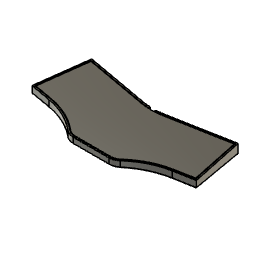
epssp75 case one-piece (Autodesk Fusion 360 design; units mm, degrees)
Autodesk Fusion 360 part; units mm, degrees
note: some values were not read from the file. Set by a fixed rule: which sketch regions a step uses.
(part 1 of 3)
sketch "Skizze1" plane through (0, 0, 0) normal (0, 0, 1) x (1, 0, 0)
  line L0 (-104.4744, 89.4694) -> (-90.6871, 87.0383)
  line L1 (-100.8347, 139.1928) -> (-114.622, 141.6239)
  line L2 (-84.0711, 124.5595) -> (-81.64, 138.3468)
  line L3 (-102.0433, 103.2567) -> (-104.4744, 89.4694)
  line L4 (-84.948, 119.5862) -> (-98.7353, 122.0173)
  line L5 (-88.256, 100.8256) -> (-102.0433, 103.2567)
  line L6 (-123.6691, 90.3154) -> (-109.8818, 87.8843)
  line L7 (-114.622, 141.6239) -> (-117.0531, 127.8365)
  line L8 (-81.64, 138.3468) -> (-95.4273, 140.7779)
  line L9 (-104.1427, 120.4322) -> (-117.93, 122.8633)
  line L10 (-107.4507, 101.6716) -> (-121.238, 104.1027)
  line L11 (-117.0531, 127.8365) -> (-103.2658, 125.4055)
  line L12 (-90.6871, 87.0383) -> (-88.256, 100.8256)
  line L13 (-97.8584, 126.9906) -> (-84.0711, 124.5595)
  line L14 (-109.8818, 87.8843) -> (-107.4507, 101.6716)
  line L15 (-103.2658, 125.4055) -> (-100.8347, 139.1928)
  line L16 (-121.238, 104.1027) -> (-123.6691, 90.3154)
  line L17 (-95.4273, 140.7779) -> (-97.8584, 126.9906)
  line L18 (-106.5738, 106.6449) -> (-104.1427, 120.4322)
  line L19 (-87.3791, 105.7989) -> (-84.948, 119.5862)
  line L20 (-98.7353, 122.0173) -> (-101.1664, 108.23)
  line L21 (-120.3611, 109.076) -> (-106.5738, 106.6449)
  line L22 (-101.1664, 108.23) -> (-87.3791, 105.7989)
  line L23 (-117.93, 122.8633) -> (-120.3611, 109.076)
  line L24 (-110.7587, 82.911) -> (-124.546, 85.3421)
  line L25 (-126.9771, 71.5548) -> (-113.1898, 69.1237)
  line L26 (-113.1898, 69.1237) -> (-110.7587, 82.911)
  line L27 (-124.546, 85.3421) -> (-126.9771, 71.5548)
  line L28 (-114.0667, 64.1504) -> (-127.854, 66.5815)
  line L29 (-130.2851, 52.7942) -> (-116.4978, 50.3631)
  line L30 (-116.4978, 50.3631) -> (-114.0667, 64.1504)
  line L31 (-127.854, 66.5815) -> (-130.2851, 52.7942)
  line L32 (-91.564, 82.065) -> (-105.3513, 84.4961)
  line L33 (-107.7824, 70.7088) -> (-93.9951, 68.2777)
  line L34 (-93.9951, 68.2777) -> (-91.564, 82.065)
  line L35 (-105.3513, 84.4961) -> (-107.7824, 70.7088)
  line L36 (-144.088, 84.2185) -> (-146.5191, 70.4311)
  line L37 (-165.2797, 73.7391) -> (-151.4924, 71.3081)
  line L38 (-154.8004, 52.5475) -> (-152.3693, 66.3348)
  line L39 (-140.78, 102.979) -> (-143.2111, 89.1917)
  line L40 (-166.1566, 68.7659) -> (-168.5877, 54.9786)
  line L41 (-126.1158, 105.5212) -> (-123.6847, 119.3086)
  line L42 (-144.8764, 108.8292) -> (-142.4453, 122.6166)
  line L43 (-168.5877, 54.9786) -> (-154.8004, 52.5475)
  line L44 (-126.9927, 100.548) -> (-140.78, 102.979)
  line L45 (-139.9031, 107.9523) -> (-126.1158, 105.5212)
  line L46 (-146.5191, 70.4311) -> (-132.7318, 68.0001)
  line L47 (-162.8486, 87.5265) -> (-165.2797, 73.7391)
  line L48 (-141.5684, 127.5898) -> (-139.1373, 141.3771)
  line L49 (-129.4238, 86.7607) -> (-126.9927, 100.548)
  line L50 (-123.6847, 119.3086) -> (-137.472, 121.7396)
  line L51 (-152.3693, 66.3348) -> (-166.1566, 68.7659)
  line L52 (-134.164, 140.5002) -> (-136.5951, 126.7129)
  line L53 (-139.1373, 141.3771) -> (-152.9246, 143.8082)
  line L54 (-136.5951, 126.7129) -> (-122.8078, 124.2818)
  line L55 (-143.2111, 89.1917) -> (-129.4238, 86.7607)
  line L56 (-158.6637, 111.2603) -> (-144.8764, 108.8292)
  line L57 (-161.9717, 92.4997) -> (-148.1844, 90.0687)
  line L58 (-149.0613, 85.0954) -> (-162.8486, 87.5265)
  line L59 (-142.4453, 122.6166) -> (-156.2326, 125.0476)
  line L60 (-148.1844, 90.0687) -> (-145.7533, 103.856)
  line L61 (-120.3767, 138.0691) -> (-134.164, 140.5002)
  line L62 (-155.3557, 130.0209) -> (-141.5684, 127.5898)
  line L63 (-156.2326, 125.0476) -> (-158.6637, 111.2603)
  line L64 (-137.472, 121.7396) -> (-139.9031, 107.9523)
  line L65 (-152.9246, 143.8082) -> (-155.3557, 130.0209)
  line L66 (-145.7533, 103.856) -> (-159.5406, 106.287)
  line L67 (-122.8078, 124.2818) -> (-120.3767, 138.0691)
  line L68 (-159.5406, 106.287) -> (-161.9717, 92.4997)
  line L69 (-132.7318, 68.0001) -> (-130.3007, 81.7874)
  line L70 (-151.4924, 71.3081) -> (-149.0613, 85.0954)
  line L71 (-130.3007, 81.7874) -> (-144.088, 84.2185)
  line L72 (-149.8271, 51.6706) -> (-136.0398, 49.2395)
  line L73 (-136.0398, 49.2395) -> (-133.6087, 63.0268)
  line L74 (-147.396, 65.4579) -> (-149.8271, 51.6706)
  line L75 (-133.6087, 63.0268) -> (-147.396, 65.4579)
  line L76 (-43.5823, 105.692) -> (-46.0133, 91.9047)
  line L77 (-28.918, 108.2342) -> (-26.4869, 122.0216)
  line L78 (-29.7949, 103.261) -> (-43.5823, 105.692)
  line L79 (-46.0133, 91.9047) -> (-32.226, 89.4737)
  line L80 (-42.7053, 110.6653) -> (-28.918, 108.2342)
  line L81 (-66.6215, 113.8162) -> (-80.4088, 116.2473)
  line L82 (-47.3313, 113.5119) -> (-44.9002, 127.2992)
  line L83 (-48.2082, 108.5386) -> (-61.9955, 110.9697)
  line L84 (-58.6875, 129.7302) -> (-61.1186, 115.9429)
  line L85 (-44.9002, 127.2992) -> (-58.6875, 129.7302)
  line L86 (-80.4088, 116.2473) -> (-82.8399, 102.46)
  line L87 (-32.226, 89.4737) -> (-29.7949, 103.261)
  line L88 (-69.0526, 100.0289) -> (-66.6215, 113.8162)
  line L89 (-64.4266, 97.1823) -> (-50.6393, 94.7513)
  line L90 (-82.8399, 102.46) -> (-69.0526, 100.0289)
  line L91 (-26.4869, 122.0216) -> (-40.2743, 124.4526)
  line L92 (-69.9295, 95.0556) -> (-83.7168, 97.4867)
  line L93 (-61.1186, 115.9429) -> (-47.3313, 113.5119)
  line L94 (-65.7446, 118.7895) -> (-63.3135, 132.5768)
  line L95 (-77.1008, 135.0079) -> (-79.5319, 121.2205)
  line L96 (-40.2743, 124.4526) -> (-42.7053, 110.6653)
  line L97 (-61.9955, 110.9697) -> (-64.4266, 97.1823)
  line L98 (-51.5162, 89.778) -> (-65.3035, 92.2091)
  line L99 (-63.3135, 132.5768) -> (-77.1008, 135.0079)
  line L100 (-79.5319, 121.2205) -> (-65.7446, 118.7895)
  line L101 (-50.6393, 94.7513) -> (-48.2082, 108.5386)
  line L102 (-83.7168, 97.4867) -> (-86.1479, 83.6994)
  line L103 (-68.6115, 73.4485) -> (-71.0426, 59.6612)
  line L104 (-72.3606, 81.2683) -> (-69.9295, 95.0556)
  line L105 (-57.2553, 57.2301) -> (-54.8242, 71.0174)
  line L106 (-86.1479, 83.6994) -> (-72.3606, 81.2683)
  line L107 (-53.9473, 75.9907) -> (-51.5162, 89.778)
  line L108 (-75.6686, 62.5077) -> (-73.2375, 76.295)
  line L109 (-54.8242, 71.0174) -> (-68.6115, 73.4485)
  line L110 (-65.3035, 92.2091) -> (-67.7346, 78.4218)
  line L111 (-67.7346, 78.4218) -> (-53.9473, 75.9907)
  line L112 (-71.0426, 59.6612) -> (-57.2553, 57.2301)
  line L113 (-87.0248, 78.7261) -> (-89.4559, 64.9388)
  line L114 (-73.2375, 76.295) -> (-87.0248, 78.7261)
  line L115 (-89.4559, 64.9388) -> (-75.6686, 62.5077)
  line L116 (-40.548, 85.3816) -> (-40.6913, 84.5691)
  line L117 (-38.9005, 60.0862) -> (-42.0814, 60.6471)
  line L118 (-43.9157, 76.735) -> (-48.5442, 77.5512)
  line L119 (-51.8862, 57.2734) -> (-52.1858, 55.5746)
  line L120 (-43.3968, 53.1872) -> (-43.2536, 53.9996)
  line L121 (-39.1207, 77.4381) -> (-35.9398, 76.8772)
  line L122 (-53.068, 57.4818) -> (-51.8862, 57.2734)
  line L123 (-34.7569, 75.1201) -> (-39.3855, 75.9362)
  line L124 (-46.6115, 61.4459) -> (-51.0136, 62.2221)
  line L125 (-40.0726, 53.4388) -> (-38.9005, 60.0862)
  line L126 (-43.6508, 78.2368) -> (-43.9157, 76.735)
  line L127 (-37.188, 61.3328) -> (-34.7569, 75.1201)
  line L128 (-48.9352, 80.9202) -> (-47.7534, 80.7118)
  line L129 (-48.0529, 79.0131) -> (-43.6508, 78.2368)
  line L130 (-50.9753, 63.7639) -> (-46.3467, 62.9477)
  line L131 (-43.2536, 53.9996) -> (-40.0726, 53.4388)
  line L132 (-41.8166, 62.1489) -> (-37.188, 61.3328)
  line L133 (-45.9962, 54.4833) -> (-46.1395, 53.6708)
  line L134 (-37.9486, 84.0855) -> (-37.8053, 84.898)
  line L135 (-35.9398, 76.8772) -> (-34.7677, 83.5246)
  line L136 (-47.1803, 83.9617) -> (-48.3621, 84.1701)
  line L137 (-34.7677, 83.5246) -> (-37.9486, 84.0855)
  line L138 (-37.8053, 84.898) -> (-40.548, 85.3816)
  line L139 (-51.0136, 62.2221) -> (-51.3132, 60.5233)
  line L140 (-39.3855, 75.9362) -> (-39.1207, 77.4381)
  line L141 (-46.1395, 53.6708) -> (-43.3968, 53.1872)
  line L142 (-48.5442, 77.5512) -> (-50.9753, 63.7639)
  line L143 (-46.8808, 85.6605) -> (-47.1803, 83.9617)
  line L144 (-52.1858, 55.5746) -> (-45.9962, 54.4833)
  line L145 (-48.3621, 84.1701) -> (-48.9352, 80.9202)
  line L146 (-42.0814, 60.6471) -> (-41.8166, 62.1489)
  line L147 (-52.4949, 60.7317) -> (-53.068, 57.4818)
  line L148 (-46.3467, 62.9477) -> (-46.6115, 61.4459)
  line L149 (-51.3132, 60.5233) -> (-52.4949, 60.7317)
  line L150 (-47.7534, 80.7118) -> (-48.0529, 79.0131)
  line L151 (-40.6913, 84.5691) -> (-46.8808, 85.6605)
  line L152 (0, 1.75) -> (0, 22.5)
  line L153 (15.275, 92.8) -> (16.1, 92.8)
  line L154 (8.525, 89.57) -> (15.275, 89.57)
  line L155 (13.55, 103.07) -> (10.25, 103.07)
  line L156 (-7, 88.1) -> (7, 88.1)
  line L157 (10.25, 101.87) -> (8.525, 101.87)
  line L158 (16.1, 92.8) -> (16.1, 95.585)
  line L159 (15.275, 101.87) -> (13.55, 101.87)
  line L160 (13.55, 101.87) -> (13.55, 103.07)
  line L161 (16.1, 95.585) -> (15.275, 95.585)
  line L162 (7, 88.1) -> (7, 92.8)
  line L163 (15.275, 95.585) -> (15.275, 101.87)
  line L164 (10.25, 103.07) -> (10.25, 101.87)
  line L165 (8.525, 101.87) -> (8.525, 97.4)
  line L166 (15.275, 89.57) -> (15.275, 92.8)
  line L167 (7, 97.4) -> (7, 102.1)
  line L168 (7, 92.8) -> (8.525, 92.8)
  line L169 (8.525, 92.8) -> (8.525, 89.57)
  line L170 (8.525, 97.4) -> (7, 97.4)
  line L171 (-8.525, 89.57) -> (-8.525, 92.8)
  line L172 (-7, 92.8) -> (-7, 88.1)
  line L173 (-16.1, 95.585) -> (-16.1, 92.8)
  line L174 (-15.275, 92.8) -> (-15.275, 89.57)
  line L175 (-7, 97.4) -> (-8.525, 97.4)
  line L176 (-15.275, 95.585) -> (-16.1, 95.585)
  line L177 (-15.275, 89.57) -> (-8.525, 89.57)
  line L178 (-8.525, 92.8) -> (-7, 92.8)
  line L179 (-10.25, 101.87) -> (-10.25, 103.07)
  line L180 (-13.55, 103.07) -> (-13.55, 101.87)
  line L181 (-8.525, 101.87) -> (-10.25, 101.87)
  line L182 (-13.55, 101.87) -> (-15.275, 101.87)
  line L183 (-15.275, 101.87) -> (-15.275, 95.585)
  line L184 (-8.525, 97.4) -> (-8.525, 101.87)
  line L185 (-10.25, 103.07) -> (-13.55, 103.07)
  line L186 (-7, 102.1) -> (-7, 97.4)
  line L187 (7, 102.1) -> (-7, 102.1)
  line L188 (-16.1, 92.8) -> (-15.275, 92.8)
  line L189 (-2.525, 121.15) -> (-16.525, 121.15)
  line L190 (-16.525, 121.15) -> (-16.525, 107.15)
  line L191 (-16.525, 107.15) -> (-2.525, 107.15)
  line L192 (-2.525, 107.15) -> (-2.525, 121.15)
  line L193 (16.525, 107.15) -> (16.525, 121.15)
  line L194 (2.525, 107.15) -> (16.525, 107.15)
  line L195 (16.525, 121.15) -> (2.525, 121.15)
  line L196 (2.525, 121.15) -> (2.525, 107.15)
  line L197 (7, 83.05) -> (-7, 83.05)
  line L198 (12.05, 83.05) -> (12.05, 69.05)
  line L199 (26.05, 69.05) -> (26.05, 83.05)
  line L200 (-7, 69.05) -> (7, 69.05)
  line L201 (12.05, 69.05) -> (26.05, 69.05)
  line L202 (-7, 83.05) -> (-7, 69.05)
  line L203 (7, 69.05) -> (7, 83.05)
  line L204 (26.05, 83.05) -> (12.05, 83.05)
  line L205 (-12.05, 83.05) -> (-26.05, 83.05)
  line L206 (-12.05, 69.05) -> (-12.05, 83.05)
  line L207 (-26.05, 83.05) -> (-26.05, 69.05)
  line L208 (-26.05, 69.05) -> (-12.05, 69.05)
  line L209 (-26.05, 50) -> (-12.05, 50)
  line L210 (-12.05, 64) -> (-26.05, 64)
  line L211 (-12.05, 50) -> (-12.05, 64)
  line L212 (7, 64) -> (-7, 64)
  line L213 (-26.05, 64) -> (-26.05, 50)
  line L214 (-7, 64) -> (-7, 50)
  line L215 (26.05, 64) -> (12.05, 64)
  line L216 (7, 50) -> (7, 64)
  line L217 (12.05, 50) -> (26.05, 50)
  line L218 (26.05, 50) -> (26.05, 64)
  line L219 (12.05, 64) -> (12.05, 50)
  line L220 (-7, 50) -> (7, 50)
  line L221 (-108.7367, 55.9946) -> (-113.525, 42.8389)
  line L222 (-95.581, 51.2064) -> (-108.7367, 55.9946)
  line L223 (-100.3693, 38.0507) -> (-95.581, 51.2064)
  line L224 (-113.525, 42.8389) -> (-100.3693, 38.0507)
  line L225 (-64.2085, 29.3272) -> (-62.5935, 32.1245)
  line L226 (-62.5935, 32.1245) -> (-61.879, 31.712)
  line L227 (-87.658, 49.8113) -> (-88.3725, 50.2238)
  line L228 (-89.765, 47.812) -> (-89.0505, 47.3995)
  line L229 (-84.8199, 41.2272) -> (-83.2049, 44.0245)
  line L230 (-68.4391, 35.4995) -> (-70.0541, 32.7022)
  line L231 (-84.2342, 39.1916) -> (-72.1098, 32.1916)
  line L232 (-90.6655, 44.6022) -> (-84.8199, 41.2272)
  line L233 (-88.3725, 50.2238) -> (-89.765, 47.812)
  line L234 (-60.4865, 34.1238) -> (-61.201, 34.5363)
  line L235 (-77.2342, 51.316) -> (-79.5842, 47.2457)
  line L236 (-58.0585, 39.9793) -> (-59.5523, 40.8418)
  line L237 (-59.5523, 40.8418) -> (-58.9523, 41.881)
  line L238 (-63.9041, 43.3543) -> (-66.1391, 39.4832)
  line L239 (-79.5638, 53.781) -> (-82.4216, 55.431)
  line L240 (-81.8842, 43.262) -> (-84.2342, 39.1916)
  line L241 (-80.9049, 48.0082) -> (-78.6699, 51.8793)
  line L242 (-58.9523, 41.881) -> (-61.8102, 43.531)
  line L243 (-82.4216, 55.431) -> (-83.0216, 54.3918)
  line L244 (-80.1638, 52.7418) -> (-79.5638, 53.781)
  line L245 (-65.1098, 44.316) -> (-77.2342, 51.316)
  line L246 (-79.5842, 47.2457) -> (-80.9049, 48.0082)
  line L247 (-89.0505, 47.3995) -> (-90.6655, 44.6022)
  line L248 (-61.201, 34.5363) -> (-58.0585, 39.9793)
  line L249 (-69.7598, 36.262) -> (-68.4391, 35.4995)
  line L250 (-83.0216, 54.3918) -> (-84.5155, 55.2543)
  line L251 (-66.1391, 39.4832) -> (-67.4598, 40.2457)
  line L252 (-70.0541, 32.7022) -> (-64.2085, 29.3272)
  line L253 (-78.6699, 51.8793) -> (-80.1638, 52.7418)
  line L254 (-83.2049, 44.0245) -> (-81.8842, 43.262)
  line L255 (-62.4102, 42.4918) -> (-63.9041, 43.3543)
  line L256 (-61.879, 31.712) -> (-60.4865, 34.1238)
  line L257 (-67.4598, 40.2457) -> (-65.1098, 44.316)
  line L258 (-61.8102, 43.531) -> (-62.4102, 42.4918)
  line L259 (-84.5155, 55.2543) -> (-87.658, 49.8113)
  line L260 (-72.1098, 32.1916) -> (-69.7598, 36.262)
  line L261 (-45.8723, 40.1216) -> (-42.448, 37.2484)
  line L262 (-36.3041, 30.1022) -> (-39.9045, 33.1233)
  line L263 (-42.448, 37.2484) -> (-43.4283, 36.0802)
  line L264 (-41.5335, 45.2924) -> (-42.6423, 43.971)
  line L265 (-36.7189, 41.2525) -> (-41.5335, 45.2924)
  line L266 (-44.7635, 41.4431) -> (-45.8723, 40.1216)
  line L267 (-42.6423, 43.971) -> (-43.5615, 44.7424)
  line L268 (-34.0551, 40.0943) -> (-36.1886, 41.8845)
  line L269 (-36.4499, 32.2153) -> (-32.1111, 37.3861)
  line L270 (-32.1111, 37.3861) -> (-34.5854, 39.4624)
  line L271 (-39.9045, 33.1233) -> (-38.9242, 34.2916)
  line L272 (-45.6827, 42.2144) -> (-44.7635, 41.4431)
  line L273 (-38.9242, 34.2916) -> (-36.4499, 32.2153)
  line L274 (-56.8318, 27.0606) -> (-57.9406, 25.7392)
  line L275 (-48.9035, 22.3987) -> (-45.3031, 19.3776)
  line L276 (-60.0618, 23.2112) -> (-61.1706, 21.8898)
  line L277 (-57.9406, 25.7392) -> (-58.8599, 26.5105)
  line L278 (-61.1706, 21.8898) -> (-56.356, 17.8499)
  line L279 (-56.356, 17.8499) -> (-56.8863, 17.2179)
  line L280 (-53.4076, 24.1873) -> (-56.8318, 27.0606)
  line L281 (-56.0277, 28.3766) -> (-52.4273, 25.3555)
  line L282 (-56.8863, 17.2179) -> (-54.7529, 15.4277)
  line L283 (-58.8599, 26.5105) -> (-60.9811, 23.9825)
  line L284 (-51.7483, 13.9835) -> (-47.4094, 19.1543)
  line L285 (-54.2226, 16.0597) -> (-51.7483, 13.9835)
  line L286 (-47.4094, 19.1543) -> (-49.8838, 21.2305)
  line L287 (-49.8838, 21.2305) -> (-48.9035, 22.3987)
  line L288 (-60.9811, 23.9825) -> (-60.0618, 23.2112)
  line L289 (-47.0287, 39.1013) -> (-56.0277, 28.3766)
  line L290 (-45.3031, 19.3776) -> (-36.3041, 30.1022)
  line L291 (-52.4273, 25.3555) -> (-53.4076, 24.1873)
  line L292 (-54.7529, 15.4277) -> (-54.2226, 16.0597)
  line L293 (-43.4283, 36.0802) -> (-47.0287, 39.1013)
  line L294 (-36.1886, 41.8845) -> (-36.7189, 41.2525)
  line L295 (-43.5615, 44.7424) -> (-45.6827, 42.2144)
  line L296 (-34.5854, 39.4624) -> (-34.0551, 40.0943)
  line L297 (-16.525, 121.15) -> (-26.4869, 122.0216) construction
  line L298 (-110.6161, 56.6787) -> (-115.4044, 43.523) construction
  line L299 (-93.7016, 50.5223) -> (-98.4899, 37.3666) construction
  line L300 (-108.7367, 55.9946) -> (-100.3693, 38.0507) construction
  line L301 (-95.581, 51.2064) -> (-113.525, 42.8389) construction
  line L302 (-77.2342, 51.316) -> (-72.1098, 32.1916) construction
  line L303 (-65.1098, 44.316) -> (-84.2342, 39.1916) construction
  line L304 (-104.553, 47.0226) -> (-74.672, 41.7538) construction
  line L305 (-57.5598, 29.6622) -> (-62.8789, 23.3232) construction
  line L306 (-35.2184, 60.9855) -> (-37.224, 49.611) construction
  line L307 (-37.224, 49.611) -> (-43.8222, 50.7744) construction
  line L308 (-48.5608, 40.3868) -> (-41.1366, 49.2346) construction
  line L309 (-41.1366, 49.2346) -> (-39.4283, 47.8012) construction
  line L310 (89.4559, 64.9388) -> (75.6686, 62.5077)
  line L311 (47.7534, 80.7118) -> (48.0529, 79.0131)
  line L312 (53.9473, 75.9907) -> (51.5162, 89.778)
  line L313 (73.2375, 76.295) -> (87.0248, 78.7261)
  line L314 (93.9951, 68.2777) -> (91.564, 82.065)
  line L315 (54.8242, 71.0174) -> (68.6115, 73.4485)
  line L316 (50.9753, 63.7639) -> (46.3467, 62.9477)
  line L317 (48.3621, 84.1701) -> (48.9352, 80.9202)
  line L318 (43.9157, 76.735) -> (48.5442, 77.5512)
  line L319 (47.1803, 83.9617) -> (48.3621, 84.1701)
  line L320 (65.7446, 118.7895) -> (63.3135, 132.5768)
  line L321 (58.6875, 129.7302) -> (61.1186, 115.9429)
  line L322 (69.0526, 100.0289) -> (66.6215, 113.8162)
  line L323 (79.5319, 121.2205) -> (65.7446, 118.7895)
  line L324 (42.7053, 110.6653) -> (28.918, 108.2342)
  line L325 (61.1186, 115.9429) -> (47.3313, 113.5119)
  line L326 (29.7949, 103.261) -> (43.5823, 105.692)
  line L327 (64.4266, 97.1823) -> (50.6393, 94.7513)
  line L328 (40.2743, 124.4526) -> (42.7053, 110.6653)
  line L329 (44.9002, 127.2992) -> (58.6875, 129.7302)
  line L330 (43.5823, 105.692) -> (46.0133, 91.9047)
  line L331 (48.2082, 108.5386) -> (61.9955, 110.9697)
  line L332 (50.6393, 94.7513) -> (48.2082, 108.5386)
  line L333 (77.1008, 135.0079) -> (79.5319, 121.2205)
  line L334 (61.9955, 110.9697) -> (64.4266, 97.1823)
  line L335 (66.6215, 113.8162) -> (80.4088, 116.2473)
  line L336 (84.0711, 124.5595) -> (81.64, 138.3468)
  line L337 (47.3313, 113.5119) -> (44.9002, 127.2992)
  line L338 (81.64, 138.3468) -> (95.4273, 140.7779)
  line L339 (69.9295, 95.0556) -> (83.7168, 97.4867)
  line L340 (82.8399, 102.46) -> (69.0526, 100.0289)
  line L341 (80.4088, 116.2473) -> (82.8399, 102.46)
  line L342 (87.3791, 105.7989) -> (84.948, 119.5862)
  line L343 (63.3135, 132.5768) -> (77.1008, 135.0079)
  line L344 (38.9005, 60.0862) -> (42.0814, 60.6471)
  line L345 (41.1366, 49.2346) -> (39.4283, 47.8012) construction
  line L346 (43.3968, 53.1872) -> (43.2536, 53.9996)
  line L347 (52.4949, 60.7317) -> (53.068, 57.4818)
  line L348 (61.8102, 43.531) -> (62.4102, 42.4918)
  line L349 (42.6423, 43.971) -> (43.5615, 44.7424)
  line L350 (45.8723, 40.1216) -> (42.448, 37.2484)
  line L351 (61.879, 31.712) -> (60.4865, 34.1238)
  line L352 (51.8862, 57.2734) -> (52.1858, 55.5746)
  line L353 (43.2536, 53.9996) -> (40.0726, 53.4388)
  line L354 (43.5615, 44.7424) -> (45.6827, 42.2144)
  line L355 (97.8584, 126.9906) -> (84.0711, 124.5595)
  line L356 (84.948, 119.5862) -> (98.7353, 122.0173)
  line L357 (46.1395, 53.6708) -> (43.3968, 53.1872)
  line L358 (40.0726, 53.4388) -> (38.9005, 60.0862)
  line L359 (45.9962, 54.4833) -> (46.1395, 53.6708)
  line L360 (95.4273, 140.7779) -> (97.8584, 126.9906)
  line L361 (53.068, 57.4818) -> (51.8862, 57.2734)
  line L362 (88.256, 100.8256) -> (102.0433, 103.2567)
  line L363 (91.564, 82.065) -> (105.3513, 84.4961)
  line L364 (51.3132, 60.5233) -> (52.4949, 60.7317)
  line L365 (52.1858, 55.5746) -> (45.9962, 54.4833)
  line L366 (52.4273, 25.3555) -> (53.4076, 24.1873)
  line L367 (44.7635, 41.4431) -> (45.8723, 40.1216)
  line L368 (59.5523, 40.8418) -> (58.9523, 41.881)
  line L369 (58.8599, 26.5105) -> (60.9811, 23.9825)
  line L370 (53.4076, 24.1873) -> (56.8318, 27.0606)
  line L371 (39.9045, 33.1233) -> (38.9242, 34.2916)
  line L372 (57.5598, 29.6622) -> (62.8789, 23.3232) construction
  line L373 (47.0287, 39.1013) -> (56.0277, 28.3766)
  line L374 (80.1638, 52.7418) -> (79.5638, 53.781)
  line L375 (90.6655, 44.6022) -> (84.8199, 41.2272)
  line L376 (87.658, 49.8113) -> (88.3725, 50.2238)
  line L377 (48.5608, 40.3868) -> (41.1366, 49.2346) construction
  line L378 (62.4102, 42.4918) -> (63.9041, 43.3543)
  line L379 (66.1391, 39.4832) -> (67.4598, 40.2457)
  line L380 (82.4216, 55.431) -> (83.0216, 54.3918)
  line L381 (43.4283, 36.0802) -> (47.0287, 39.1013)
  line L382 (56.0277, 28.3766) -> (52.4273, 25.3555)
  line L383 (62.5935, 32.1245) -> (61.879, 31.712)
  line L384 (65.1098, 44.316) -> (77.2342, 51.316)
  line L385 (41.5335, 45.2924) -> (42.6423, 43.971)
  line L386 (56.8318, 27.0606) -> (57.9406, 25.7392)
  line L387 (78.6699, 51.8793) -> (80.1638, 52.7418)
  line L388 (67.4598, 40.2457) -> (65.1098, 44.316)
  line L389 (42.448, 37.2484) -> (43.4283, 36.0802)
  line L390 (60.4865, 34.1238) -> (61.201, 34.5363)
  line L391 (64.2085, 29.3272) -> (62.5935, 32.1245)
  line L392 (57.9406, 25.7392) -> (58.8599, 26.5105)
  line L393 (61.201, 34.5363) -> (58.0585, 39.9793)
  line L394 (89.0505, 47.3995) -> (90.6655, 44.6022)
  line L395 (79.5638, 53.781) -> (82.4216, 55.431)
  line L396 (58.0585, 39.9793) -> (59.5523, 40.8418)
  line L397 (60.9811, 23.9825) -> (60.0618, 23.2112)
  line L398 (89.765, 47.812) -> (89.0505, 47.3995)
  line L399 (88.3725, 50.2238) -> (89.765, 47.812)
  line L400 (45.6827, 42.2144) -> (44.7635, 41.4431)
  line L401 (58.9523, 41.881) -> (61.8102, 43.531)
  line L402 (123.6691, 90.3154) -> (109.8818, 87.8843)
  line L403 (113.1898, 69.1237) -> (110.7587, 82.911)
  line L404 (51.5162, 89.778) -> (65.3035, 92.2091)
  line L405 (114.0667, 64.1504) -> (127.854, 66.5815)
  line L406 (161.9717, 92.4997) -> (148.1844, 90.0687)
  line L407 (126.1158, 105.5212) -> (123.6847, 119.3086)
  line L408 (90.6871, 87.0383) -> (88.256, 100.8256)
  line L409 (132.7318, 68.0001) -> (130.3007, 81.7874)
  line L410 (102.0433, 103.2567) -> (104.4744, 89.4694)
  line L411 (151.4924, 71.3081) -> (149.0613, 85.0954)
  line L412 (149.0613, 85.0954) -> (162.8486, 87.5265)
  line L413 (126.9771, 71.5548) -> (113.1898, 69.1237)
  line L414 (133.6087, 63.0268) -> (147.396, 65.4579)
  line L415 (105.3513, 84.4961) -> (107.7824, 70.7088)
  line L416 (165.2797, 73.7391) -> (151.4924, 71.3081)
  line L417 (109.8818, 87.8843) -> (107.4507, 101.6716)
  line L418 (146.5191, 70.4311) -> (132.7318, 68.0001)
  line L419 (46.0133, 91.9047) -> (32.226, 89.4737)
  line L420 (124.546, 85.3421) -> (126.9771, 71.5548)
  line L421 (65.3035, 92.2091) -> (67.7346, 78.4218)
  line L422 (120.3767, 138.0691) -> (134.164, 140.5002)
  line L423 (126.9927, 100.548) -> (140.78, 102.979)
  line L424 (141.5684, 127.5898) -> (139.1373, 141.3771)
  line L425 (130.3007, 81.7874) -> (144.088, 84.2185)
  line L426 (83.7168, 97.4867) -> (86.1479, 83.6994)
  line L427 (148.1844, 90.0687) -> (145.7533, 103.856)
  line L428 (140.78, 102.979) -> (143.2111, 89.1917)
  line L429 (122.8078, 124.2818) -> (120.3767, 138.0691)
  line L430 (32.226, 89.4737) -> (29.7949, 103.261)
  line L431 (72.3606, 81.2683) -> (69.9295, 95.0556)
  line L432 (110.7587, 82.911) -> (124.546, 85.3421)
  line L433 (143.2111, 89.1917) -> (129.4238, 86.7607)
  line L434 (152.3693, 66.3348) -> (166.1566, 68.7659)
  line L435 (144.088, 84.2185) -> (146.5191, 70.4311)
  line L436 (162.8486, 87.5265) -> (165.2797, 73.7391)
  line L437 (129.4238, 86.7607) -> (126.9927, 100.548)
  line L438 (37.188, 61.3328) -> (34.7569, 75.1201)
  line L439 (61.1706, 21.8898) -> (56.356, 17.8499)
  line L440 (68.6115, 73.4485) -> (71.0426, 59.6612)
  line L441 (166.1566, 68.7659) -> (168.5877, 54.9786)
  line L442 (113.525, 42.8389) -> (100.3693, 38.0507)
  line L443 (168.5877, 54.9786) -> (154.8004, 52.5475)
  line L444 (154.8004, 52.5475) -> (152.3693, 66.3348)
  line L445 (45.3031, 19.3776) -> (36.3041, 30.1022)
  line L446 (48.9035, 22.3987) -> (45.3031, 19.3776)
  line L447 (147.396, 65.4579) -> (149.8271, 51.6706)
  line L448 (49.8838, 21.2305) -> (48.9035, 22.3987)
  line L449 (93.7016, 50.5223) -> (98.4899, 37.3666) construction
  line L450 (56.356, 17.8499) -> (56.8863, 17.2179)
  line L451 (127.854, 66.5815) -> (130.2851, 52.7942)
  line L452 (56.8863, 17.2179) -> (54.7529, 15.4277)
  line L453 (104.553, 47.0226) -> (74.672, 41.7538) construction
  line L454 (51.0136, 62.2221) -> (51.3132, 60.5233)
  line L455 (110.6161, 56.6787) -> (115.4044, 43.523) construction
  line L456 (46.3467, 62.9477) -> (46.6115, 61.4459)
  line L457 (54.2226, 16.0597) -> (51.7483, 13.9835)
  line L458 (46.6115, 61.4459) -> (51.0136, 62.2221)
  line L459 (100.3693, 38.0507) -> (95.581, 51.2064)
  line L460 (95.581, 51.2064) -> (108.7367, 55.9946)
  line L461 (108.7367, 55.9946) -> (100.3693, 38.0507) construction
  line L462 (42.0814, 60.6471) -> (41.8166, 62.1489)
  line L463 (136.0398, 49.2395) -> (133.6087, 63.0268)
  line L464 (116.4978, 50.3631) -> (114.0667, 64.1504)
  line L465 (47.4094, 19.1543) -> (49.8838, 21.2305)
  line L466 (60.0618, 23.2112) -> (61.1706, 21.8898)
  line L467 (149.8271, 51.6706) -> (136.0398, 49.2395)
  line L468 (130.2851, 52.7942) -> (116.4978, 50.3631)
  line L469 (108.7367, 55.9946) -> (113.525, 42.8389)
  line L470 (95.581, 51.2064) -> (113.525, 42.8389) construction
  line L471 (57.2553, 57.2301) -> (54.8242, 71.0174)
  line L472 (41.8166, 62.1489) -> (37.188, 61.3328)
  line L473 (51.7483, 13.9835) -> (47.4094, 19.1543)
  line L474 (54.7529, 15.4277) -> (54.2226, 16.0597)
  line L475 (84.8199, 41.2272) -> (83.2049, 44.0245)
  line L476 (36.7189, 41.2525) -> (41.5335, 45.2924)
  line L477 (34.5854, 39.4624) -> (34.0551, 40.0943)
  line L478 (84.5155, 55.2543) -> (87.658, 49.8113)
  line L479 (72.1098, 32.1916) -> (69.7598, 36.262)
  line L480 (77.2342, 51.316) -> (72.1098, 32.1916) construction
  line L481 (70.0541, 32.7022) -> (64.2085, 29.3272)
  line L482 (71.0426, 59.6612) -> (57.2553, 57.2301)
  line L483 (32.1111, 37.3861) -> (34.5854, 39.4624)
  line L484 (77.2342, 51.316) -> (79.5842, 47.2457)
  line L485 (63.9041, 43.3543) -> (66.1391, 39.4832)
  line L486 (83.2049, 44.0245) -> (81.8842, 43.262)
  line L487 (79.5842, 47.2457) -> (80.9049, 48.0082)
  line L488 (68.4391, 35.4995) -> (70.0541, 32.7022)
  line L489 (34.0551, 40.0943) -> (36.1886, 41.8845)
  line L490 (36.1886, 41.8845) -> (36.7189, 41.2525)
  line L491 (36.3041, 30.1022) -> (39.9045, 33.1233)
  line L492 (80.9049, 48.0082) -> (78.6699, 51.8793)
  line L493 (81.8842, 43.262) -> (84.2342, 39.1916)
  line L494 (36.4499, 32.2153) -> (32.1111, 37.3861)
  line L495 (37.224, 49.611) -> (43.8222, 50.7744) construction
  line L496 (69.7598, 36.262) -> (68.4391, 35.4995)
  line L497 (83.0216, 54.3918) -> (84.5155, 55.2543)
  line L498 (84.2342, 39.1916) -> (72.1098, 32.1916)
  line L499 (35.2184, 60.9855) -> (37.224, 49.611) construction
  line L500 (38.9242, 34.2916) -> (36.4499, 32.2153)
  line L501 (65.1098, 44.316) -> (84.2342, 39.1916) construction
  line L502 (40.6913, 84.5691) -> (46.8808, 85.6605)
  line L503 (43.6508, 78.2368) -> (43.9157, 76.735)
  line L504 (34.7677, 83.5246) -> (37.9486, 84.0855)
  line L505 (86.1479, 83.6994) -> (72.3606, 81.2683)
  line L506 (87.0248, 78.7261) -> (89.4559, 64.9388)
  line L507 (75.6686, 62.5077) -> (73.2375, 76.295)
  line L508 (48.9352, 80.9202) -> (47.7534, 80.7118)
  line L509 (48.5442, 77.5512) -> (50.9753, 63.7639)
  line L510 (39.3855, 75.9362) -> (39.1207, 77.4381)
  line L511 (37.8053, 84.898) -> (40.548, 85.3816)
  line L512 (37.9486, 84.0855) -> (37.8053, 84.898)
  line L513 (46.8808, 85.6605) -> (47.1803, 83.9617)
  line L514 (40.548, 85.3816) -> (40.6913, 84.5691)
  line L515 (48.0529, 79.0131) -> (43.6508, 78.2368)
  line L516 (34.7569, 75.1201) -> (39.3855, 75.9362)
  line L517 (67.7346, 78.4218) -> (53.9473, 75.9907)
  line L518 (35.9398, 76.8772) -> (34.7677, 83.5246)
  line L519 (39.1207, 77.4381) -> (35.9398, 76.8772)
  line L520 (107.4507, 101.6716) -> (121.238, 104.1027)
  line L521 (134.164, 140.5002) -> (136.5951, 126.7129)
  line L522 (100.8347, 139.1928) -> (114.622, 141.6239)
  line L523 (123.6847, 119.3086) -> (137.472, 121.7396)
  line L524 (145.7533, 103.856) -> (159.5406, 106.287)
  line L525 (144.8764, 108.8292) -> (142.4453, 122.6166)
  line L526 (152.9246, 143.8082) -> (155.3557, 130.0209)
  line L527 (137.472, 121.7396) -> (139.9031, 107.9523)
  line L528 (117.93, 122.8633) -> (120.3611, 109.076)
  line L529 (98.7353, 122.0173) -> (101.1664, 108.23)
  line L530 (136.5951, 126.7129) -> (122.8078, 124.2818)
  line L531 (101.1664, 108.23) -> (87.3791, 105.7989)
  line L532 (106.5738, 106.6449) -> (104.1427, 120.4322)
  line L533 (158.6637, 111.2603) -> (144.8764, 108.8292)
  line L534 (142.4453, 122.6166) -> (156.2326, 125.0476)
  line L535 (139.9031, 107.9523) -> (126.1158, 105.5212)
  line L536 (103.2658, 125.4055) -> (100.8347, 139.1928)
  line L537 (159.5406, 106.287) -> (161.9717, 92.4997)
  line L538 (121.238, 104.1027) -> (123.6691, 90.3154)
  line L539 (156.2326, 125.0476) -> (158.6637, 111.2603)
  line L540 (114.622, 141.6239) -> (117.0531, 127.8365)
  line L541 (139.1373, 141.3771) -> (152.9246, 143.8082)
  line L542 (120.3611, 109.076) -> (106.5738, 106.6449)
  line L543 (104.4744, 89.4694) -> (90.6871, 87.0383)
  line L544 (107.7824, 70.7088) -> (93.9951, 68.2777)
  line L545 (155.3557, 130.0209) -> (141.5684, 127.5898)
  line L546 (104.1427, 120.4322) -> (117.93, 122.8633)
  line L547 (117.0531, 127.8365) -> (103.2658, 125.4055)
  line L548 (26.4869, 122.0216) -> (40.2743, 124.4526)
  line L549 (28.918, 108.2342) -> (26.4869, 122.0216)
  line L550 (-157.0019, 158.2608) -> (-24.2252, 134.8487)
  line L551 (-157.0019, 158.2608) -> (-176.1466, 49.6857)
  line L552 (-176.1466, 49.6857) -> (-132.1996, 41.9367)
  arc A0 (-56.1359, 6.4676) -> (-132.1996, 41.9367) centre (-160.3539, -117.7346) ccw
  line L553 (-56.1359, 6.4676) -> (-41.0203, -6.2159) construction
  line L554 (157.0019, 158.2608) -> (24.2252, 134.8487)
  line L555 (157.0019, 158.2608) -> (176.1466, 49.6857)
  arc A1 (132.1996, 41.9367) -> (56.1359, 6.4676) centre (160.3539, -117.7346) ccw
  line L556 (176.1466, 49.6857) -> (132.1996, 41.9367)
  line L557 (56.1359, 6.4676) -> (41.0203, -6.2159) construction
  arc A2 (-24.2252, 134.8487) -> (24.2252, 134.8487) centre (0, 272.2365) ccw
  arc A3 (-56.1359, 6.4676) -> (-38.3662, 0) centre (-38.3662, 27.6446) ccw
  line L558 (1.75, 0) -> (22.5, 0)
  arc A4 (38.3662, 0) -> (56.1359, 6.4676) centre (38.3662, 27.6446) ccw
  line L559 (-38.3662, 0) -> (38.3662, 0)
  point P0 (0, 88.1)
  point P1 (-111.1309, 49.4168)
  point P2 (-114.8755, 48.0462)
  point P3 (-104.553, 47.0226)
  point P4 (-74.672, 41.7538)
  point P5 (-95.2368, 43.2346)
  point P6 (-63.1072, 24.6846)
  point P7 (95.2368, 43.2346)
  point P8 (111.1309, 49.4168)
  point P9 (74.672, 41.7538)
  point P10 (104.553, 47.0226)
  point P11 (114.8755, 48.0462)
  point P12 (63.1072, 24.6846)
  dimension "d2" = 14
  dimension "d3" = 14
  dimension "d6" = 14
  dimension "d7" = 14
  dimension "d9" = 14
  dimension "d10" = 14
  dimension "d11" = 14
  dimension "d12" = 14
  dimension "d13" = 5.05
  dimension "d14" = 14
  dimension "d15" = 14
  dimension "d16" = 14
  dimension "d17" = 14
  dimension "d128" = 14
  dimension "d129" = 14
  dimension "d130" = 14
  dimension "d131" = 14
  dimension "d132" = 5.05
  dimension "d133" = 5.05
  dimension "d134" = 5.05
  dimension "d135" = 5.05
  dimension "d136" = 5.05
  dimension "d137" = 5.05
  dimension "d138" = 14
  dimension "d139" = 14
  dimension "d140" = 5.05
  dimension "d141" = 2.5
  dimension "d142" = 14
  dimension "d143" = 14
  dimension "d144" = 14
  dimension "d145" = 14
  dimension "d146" = 14
  dimension "d147" = 14
  dimension "d148" = 14
  dimension "d149" = 14
  dimension "d150" = 5.05
  dimension "d151" = 14
  dimension "d152" = 14
  dimension "d153" = 14
  dimension "d154" = 14
  dimension "d155" = 14
  dimension "d156" = 14
  dimension "d157" = 14
  dimension "d158" = 14
  dimension "d159" = 5.05
  dimension "d160" = 5.05
  dimension "d161" = 5.05
  dimension "d162" = 5.05
  dimension "d163" = 5.05
  dimension "d164" = 5.05
  dimension "d165" = 14
  dimension "d166" = 14
  dimension "d167" = 5.05
  dimension "d169" = 5.05
  dimension "d170" = 14
  dimension "d171" = 14
  dimension "d172" = 5.05
  dimension "d173" = 7
  dimension "d176" = 14
  dimension "d177" = 14
  dimension "d180" = 14
  dimension "d181" = 14
  dimension "d191" = 5.05
  dimension "d201" = 14
  dimension "d202" = 14
  dimension "d203" = 14
  dimension "d204" = 14
  dimension "d205" = 14
  dimension "d206" = 14
  dimension "d207" = 14
  dimension "d208" = 14
  dimension "d209" = 5.05
  dimension "d210" = 14
  dimension "d211" = 14
  dimension "d212" = 14
  dimension "d213" = 14
  dimension "d214" = 14
  dimension "d215" = 14
  dimension "d218" = 5.05
  dimension "d219" = 5.05
  dimension "d220" = 5.05
  dimension "d221" = 5.05
  dimension "d222" = 5.05
  dimension "d224" = 14
  dimension "d225" = 14
  dimension "d226" = 5.05
  dimension "d227" = 5.05
  dimension "d232" = 5.05
  dimension "d234" = 4.5
  dimension "d235" = 6.5
  dimension "d236" = 3.3
  dimension "d237" = 1.2
  dimension "d238" = 1.725
  dimension "d239" = 1.725
  dimension "d240" = 1.725
  dimension "d241" = 1.725
  dimension "d242" = 3.3
  dimension "d245" = 6.75
  dimension "d246" = 6.75
  dimension "d247" = 3.23
  dimension "d248" = 4.7
  dimension "d249" = 14
  dimension "d250" = 14
  dimension "d251" = 6.285
  dimension "d252" = 0.825
  dimension "d254" = 2.785
  dimension "d255" = 1.525
  dimension "d256" = 4.47
  dimension "d257" = 4.7
  dimension "d258" = 14.575
  dimension "d261" = 3.3
  dimension "d262" = 1.2
  dimension "d263" = 1.725
  dimension "d264" = 1.725
  dimension "d265" = 1.725
  dimension "d266" = 1.725
  dimension "d267" = 3.3
  dimension "d268" = 6.75
  dimension "d269" = 6.75
  dimension "d270" = 3.23
  dimension "d271" = 4.7
  dimension "d272" = 14
  dimension "d273" = 14
  dimension "d274" = 6.285
  dimension "d275" = 0.825
  dimension "d276" = 2.785
  dimension "d277" = 1.525
  dimension "d278" = 4.47
  dimension "d279" = 4.7
  dimension "d280" = 14
  dimension "d281" = 14
  dimension "d282" = 14
  dimension "d283" = 14
  dimension "d284" = 5.05
  dimension "d285" = 5.05
  dimension "d286" = 2.525
  dimension "d287" = 14
  dimension "d288" = 14
  dimension "d289" = 14
  dimension "d290" = 14
  dimension "d291" = 5.05
  dimension "d292" = 14
  dimension "d293" = 14
  dimension "d294" = 5.05
  dimension "d295" = 14
  dimension "d296" = 14
  dimension "d297" = 14
  dimension "d298" = 14
  dimension "d300" = 14
  dimension "d301" = 14
  dimension "d303" = 5.05
  dimension "d305" = 5.05
  dimension "d306" = 14
  dimension "d307" = 14
  dimension "d312" = 3.3
  dimension "d313" = 1.2
  dimension "d314" = 1.725
  dimension "d315" = 1.725
  dimension "d316" = 1.725
  dimension "d317" = 1.725
  dimension "d318" = 3.3
  dimension "d319" = 6.75
  dimension "d320" = 6.75
  dimension "d321" = 3.23
  dimension "d322" = 4.7
  dimension "d323" = 14
  dimension "d324" = 14
  dimension "d325" = 6.285
  dimension "d326" = 0.825
  dimension "d327" = 2.785
  dimension "d328" = 1.525
  dimension "d329" = 4.47
  dimension "d330" = 4.7
  dimension "d375" = 3.3
  dimension "d376" = 1.2
  dimension "d377" = 1.725
  dimension "d378" = 1.725
  dimension "d379" = 1.725
  dimension "d380" = 1.725
  dimension "d381" = 3.3
  dimension "d382" = 6.75
  dimension "d383" = 6.75
  dimension "d384" = 3.23
  dimension "d385" = 4.7
  dimension "d386" = 14
  dimension "d387" = 14
  dimension "d388" = 6.285
  dimension "d389" = 0.825
  dimension "d390" = 2.785
  dimension "d391" = 1.525
  dimension "d392" = 4.47
  dimension "d393" = 4.7
  dimension "d395" = 50
  dimension "d397" = 95
  dimension "d398" = 95
  dimension "d399" = 10
  dimension "d401" = 2
  dimension "d402" = 2
  dimension "d403" = 2
  dimension "d404" = 1.05
  dimension "d405" = 2
  dimension "d406" = 10
  dimension "d407" = 10
  dimension "d408" = 2
  dimension "d409" = 11.55
  dimension "d410" = 1.05
  dimension "d411" = 2
  dimension "d412" = 11.55
  dimension "d413" = 2
  dimension "d414" = 1.05
  dimension "d415" = 2
  dimension "d416" = 11.55
  dimension "d418" = 10
  dimension "d419" = 2
  dimension "d420" = 11.55
  dimension "d421" = 1.05
  dimension "d423" = 6.525
  dimension "d424" = 6.525
  dimension "d425" = 6.525
  constraint perpendicular L4 L20
  constraint perpendicular L20 L22
  constraint perpendicular L9 L23
  constraint perpendicular L21 L23
  constraint perpendicular L8 L17
  constraint perpendicular L13 L17
  constraint perpendicular L1 L7
  constraint perpendicular L7 L11
  constraint collinear L15 L18
  constraint collinear L2 L19
  constraint perpendicular L3 L5
  constraint perpendicular L0 L3
  constraint perpendicular L10 L16
  constraint perpendicular L6 L16
  constraint collinear L14 L18
  constraint collinear L12 L19
  constraint perpendicular L24 L27
  constraint perpendicular L25 L27
  constraint perpendicular L28 L31
  constraint perpendicular L29 L31
  constraint perpendicular L32 L35
  constraint perpendicular L33 L35
  constraint collinear L14 L26
  constraint collinear L26 L30
  constraint collinear L12 L34
  constraint perpendicular L2 L8
  constraint perpendicular L1 L15
  constraint perpendicular L50 L64
  constraint perpendicular L45 L64
  constraint perpendicular L59 L63
  constraint perpendicular L56 L63
  constraint perpendicular L52 L61
  constraint perpendicular L52 L54
  constraint perpendicular L53 L65
  constraint perpendicular L62 L65
  constraint collinear L42 L48
  constraint collinear L41 L67
  constraint perpendicular L39 L44
  constraint perpendicular L39 L55
  constraint perpendicular L66 L68
  constraint perpendicular L57 L68
  constraint collinear L42 L60
  constraint collinear L41 L49
  constraint perpendicular L47 L58
  constraint perpendicular L37 L47
  constraint perpendicular L40 L51
  constraint perpendicular L40 L43
  constraint perpendicular L36 L71
  constraint perpendicular L36 L46
  constraint collinear L60 L70
  constraint collinear L38 L70
  constraint collinear L49 L69
  constraint perpendicular L61 L67
  constraint perpendicular L48 L53
  constraint perpendicular L74 L75
  constraint perpendicular L72 L74
  constraint collinear L69 L73
  constraint collinear L53 L61
  constraint perpendicular L76 L78
  constraint perpendicular L76 L79
  constraint perpendicular L91 L96
  constraint perpendicular L80 L96
  constraint collinear L77 L87
  constraint perpendicular L77 L91
  constraint perpendicular L83 L97
  constraint perpendicular L89 L97
  constraint perpendicular L81 L86
  constraint perpendicular L86 L90
  constraint perpendicular L84 L85
  constraint perpendicular L84 L93
  constraint perpendicular L95 L99
  constraint perpendicular L95 L100
  constraint collinear L88 L94
  constraint collinear L82 L101
  constraint perpendicular L98 L110
  constraint perpendicular L110 L111
  constraint perpendicular L92 L102
  constraint perpendicular L102 L106
  constraint collinear L88 L104
  constraint collinear L101 L107
  constraint perpendicular L113 L114
  constraint perpendicular L113 L115
  constraint perpendicular L103 L109
  constraint perpendicular L103 L112
  constraint collinear L104 L108
  constraint collinear L105 L107
  constraint perpendicular L82 L85
  constraint perpendicular L94 L99
  constraint collinear L1 L99
  constraint perpendicular L143 L151
  constraint perpendicular L116 L151
  constraint perpendicular L116 L138
  constraint perpendicular L134 L138
  constraint perpendicular L134 L137
  constraint perpendicular L135 L137
  constraint perpendicular L121 L135
  constraint perpendicular L121 L140
  constraint perpendicular L123 L140
  constraint perpendicular L123 L127
  constraint perpendicular L127 L132
  constraint perpendicular L132 L146
  constraint perpendicular L117 L146
  constraint perpendicular L117 L125
  constraint perpendicular L125 L131
  constraint perpendicular L120 L131
  constraint perpendicular L120 L141
  constraint perpendicular L133 L141
  constraint perpendicular L133 L144
  constraint perpendicular L119 L144
  constraint perpendicular L119 L122
  constraint perpendicular L122 L147
  constraint perpendicular L147 L149
  constraint perpendicular L139 L149
  constraint perpendicular L124 L139
  constraint perpendicular L124 L148
  constraint perpendicular L130 L148
  constraint perpendicular L130 L142
  constraint perpendicular L118 L142
  constraint perpendicular L118 L126
  constraint perpendicular L126 L129
  constraint perpendicular L129 L150
  constraint perpendicular L128 L150
  constraint perpendicular L128 L145
  constraint perpendicular L136 L145
  constraint collinear L137 L151
  constraint collinear L131 L144
  constraint collinear L121 L129
  constraint collinear L118 L123
  constraint collinear L130 L132
  constraint collinear L117 L124
  constraint collinear L125 L135
  constraint collinear L119 L139
  constraint collinear L139 L150
  constraint collinear L143 L150
  constraint collinear L145 L147
  constraint collinear L140 L146
  constraint collinear L126 L148
  constraint collinear L120 L146
  constraint collinear L134 L140
  constraint collinear L116 L133
  constraint equal L116 L133
  constraint equal L140 L146
  constraint parallel L79 L151
  constraint collinear L87 L127
  constraint perpendicular L159 L163
  constraint perpendicular L161 L163
  constraint perpendicular L158 L161
  constraint perpendicular L153 L158
  constraint perpendicular L153 L166
  constraint perpendicular L154 L166
  constraint perpendicular L154 L169
  constraint perpendicular L168 L169
  constraint perpendicular L162 L168
  constraint perpendicular L156 L162
  constraint perpendicular L156 L172
  constraint perpendicular L172 L178
  constraint perpendicular L171 L178
  constraint perpendicular L171 L177
  constraint perpendicular L174 L177
  constraint perpendicular L174 L188
  constraint perpendicular L173 L188
  constraint perpendicular L173 L176
  constraint perpendicular L176 L183
  constraint perpendicular L182 L183
  constraint perpendicular L180 L182
  constraint perpendicular L180 L185
  constraint perpendicular L179 L185
  constraint perpendicular L179 L181
  constraint perpendicular L181 L184
  constraint perpendicular L175 L184
  constraint perpendicular L175 L186
  constraint perpendicular L186 L187
  constraint perpendicular L167 L187
  constraint perpendicular L167 L170
  constraint perpendicular L165 L170
  constraint perpendicular L157 L165
  constraint perpendicular L157 L164
  constraint perpendicular L155 L164
  constraint perpendicular L155 L160
  constraint collinear L163 L166
  constraint collinear L174 L183
  constraint collinear L165 L169
  constraint collinear L162 L167
  constraint collinear L172 L186
  constraint collinear L171 L184
  constraint collinear L154 L177
  constraint collinear L181 L182
  constraint collinear L157 L181
  constraint collinear L157 L159
  constraint collinear L155 L185
  constraint collinear L168 L178
  constraint collinear L170 L175
  constraint collinear L178 L188
  constraint collinear L153 L168
  constraint collinear L161 L176
  constraint equal L161 L176
  constraint equal L168 L178
  constraint midpoint L156 P0
  constraint coincident L152 P0
  constraint perpendicular L189 L190
  constraint perpendicular L190 L191
  constraint perpendicular L189 L192
  constraint perpendicular L195 L196
  constraint perpendicular L194 L196
  constraint perpendicular L193 L195
  constraint collinear L189 L195
  constraint horizontal L156
  constraint perpendicular L197 L202
  constraint perpendicular L200 L202
  constraint perpendicular L197 L203
  constraint perpendicular L198 L204
  constraint perpendicular L198 L201
  constraint perpendicular L199 L204
  constraint collinear L197 L204
  constraint perpendicular L205 L207
  constraint perpendicular L207 L208
  constraint perpendicular L205 L206
  constraint collinear L197 L205
  constraint perpendicular L212 L214
  constraint perpendicular L214 L220
  constraint perpendicular L212 L216
  constraint perpendicular L215 L219
  constraint perpendicular L217 L219
  constraint perpendicular L215 L218
  constraint collinear L212 L215
  constraint perpendicular L210 L213
  constraint perpendicular L209 L213
  constraint perpendicular L210 L211
  constraint collinear L210 L212
  constraint collinear L206 L211
  constraint collinear L198 L219
  constraint collinear L202 L214
  constraint collinear L172 L202
  constraint perpendicular L221 L222
  constraint perpendicular L221 L224
  constraint perpendicular L222 L223
  constraint perpendicular L236 L248
  constraint perpendicular L234 L248
  constraint perpendicular L234 L256
  constraint perpendicular L226 L256
  constraint perpendicular L225 L226
  constraint perpendicular L225 L252
  constraint perpendicular L230 L252
  constraint perpendicular L230 L249
  constraint perpendicular L249 L260
  constraint perpendicular L231 L260
  constraint perpendicular L231 L240
  constraint perpendicular L240 L254
  constraint perpendicular L229 L254
  constraint perpendicular L229 L232
  constraint perpendicular L232 L247
  constraint perpendicular L228 L247
  constraint perpendicular L228 L233
  constraint perpendicular L227 L233
  constraint perpendicular L227 L259
  constraint perpendicular L250 L259
  constraint perpendicular L243 L250
  constraint perpendicular L239 L243
  constraint perpendicular L239 L244
  constraint perpendicular L244 L253
  constraint perpendicular L241 L253
  constraint perpendicular L241 L246
  constraint perpendicular L235 L246
  constraint perpendicular L235 L245
  constraint perpendicular L245 L257
  constraint perpendicular L251 L257
  constraint perpendicular L238 L251
  constraint perpendicular L238 L255
  constraint perpendicular L255 L258
  constraint perpendicular L242 L258
  constraint perpendicular L237 L242
  constraint collinear L225 L248
  constraint collinear L247 L259
  constraint collinear L230 L238
  constraint collinear L257 L260
  constraint collinear L235 L240
  constraint collinear L229 L241
  constraint collinear L232 L252
  constraint collinear L250 L253
  constraint collinear L253 L255
  constraint collinear L236 L255
  constraint collinear L239 L242
  constraint collinear L249 L254
  constraint collinear L246 L251
  constraint collinear L228 L254
  constraint collinear L226 L249
  constraint collinear L227 L234
  constraint equal L227 L234
  constraint equal L249 L254
  constraint perpendicular L264 L265
  constraint perpendicular L265 L294
  constraint perpendicular L268 L294
  constraint perpendicular L268 L296
  constraint perpendicular L270 L296
  constraint perpendicular L269 L270
  constraint perpendicular L269 L273
  constraint perpendicular L271 L273
  constraint perpendicular L262 L271
  constraint perpendicular L262 L290
  constraint perpendicular L275 L290
  constraint perpendicular L275 L287
  constraint perpendicular L286 L287
  constraint perpendicular L284 L286
  constraint perpendicular L284 L285
  constraint perpendicular L285 L292
  constraint perpendicular L282 L292
  constraint perpendicular L279 L282
  constraint perpendicular L278 L279
  constraint perpendicular L276 L278
  constraint perpendicular L276 L288
  constraint perpendicular L283 L288
  constraint perpendicular L277 L283
  constraint perpendicular L274 L277
  constraint perpendicular L274 L280
  constraint perpendicular L280 L291
  constraint perpendicular L281 L291
  constraint perpendicular L281 L289
  constraint perpendicular L289 L293
  constraint perpendicular L263 L293
  constraint perpendicular L261 L263
  constraint perpendicular L261 L266
  constraint perpendicular L266 L272
  constraint perpendicular L272 L295
  constraint perpendicular L267 L295
  constraint collinear L265 L270
  constraint collinear L278 L285
  constraint collinear L261 L273
  constraint collinear L262 L293
  constraint collinear L275 L281
  constraint collinear L280 L286
  constraint collinear L269 L284
  constraint collinear L274 L276
  constraint collinear L266 L274
  constraint collinear L264 L266
  constraint collinear L283 L295
  constraint collinear L271 L287
  constraint collinear L263 L291
  constraint collinear L287 L292
  constraint collinear L271 L296
  constraint collinear L279 L294
  constraint equal L279 L294
  constraint equal L271 L287
  constraint midpoint L221 P1
  constraint coincident L29 P1
  constraint perpendicular L222 L298
  constraint coincident L222 L298.start
  constraint coincident L224 L298.end
  constraint coincident L222 L299.start
  constraint coincident L224 L299.end
  constraint perpendicular L222 L299
  constraint midpoint L301 P3
  constraint midpoint L303 P4
  constraint coincident P3 L304.start
  constraint coincident P4 L304.end
  constraint parallel L115 L304
  constraint parallel L289 L305
  constraint coincident L281 L305.start
  constraint perpendicular L117 L306
  constraint perpendicular L146 L307
  constraint coincident L132 L306.start
  constraint coincident L120 L307.end
  constraint perpendicular L272 L308
  constraint perpendicular L289 L309
  constraint coincident L293 L308.start
  constraint coincident L264 L309.end
  constraint coincident L278 L305.end
  constraint symmetric L10.start L152 L417.end
  constraint symmetric L0.end L152 L408.start
  constraint symmetric L13.start L152 L355.start
  constraint symmetric L2.end L152 L336.end
  constraint symmetric L6.start L152 L402.start
  constraint symmetric L8.end L152 L338.end
  constraint symmetric L3.start L152 L362.end
  constraint symmetric L10.end L152 L520.end